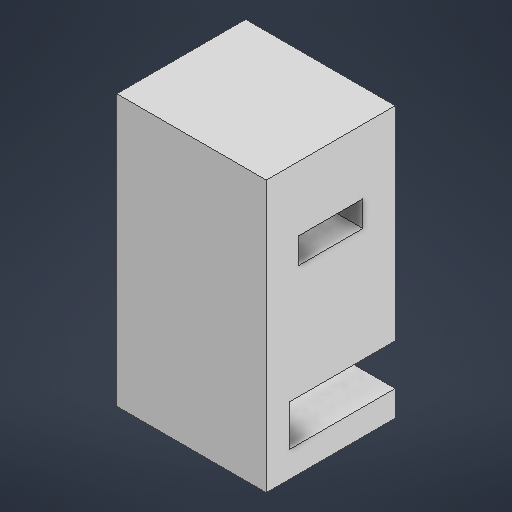
# Autodesk Inventor part: drone_battery_holder
Saved by Autodesk Inventor 2026.1 (Build 301233000, 233)
## iProperties
Created: 2025-08-09
Part Number: drone_battery_holder
Material: Generic
Document SubType Name: Modeling
Designer: rohit
Density: 1 g/cm^3
Appearance: Default
Author: rohit
Autodesk Inventor part; units mm, degrees
ref_plane "YZ Plane" through (0, 0, 0) normal (1, 0, 0) x (0, 1, 0)
ref_plane "XZ Plane" through (0, 0, 0) normal (0, 1, 0) x (-1, 0, 0)
ref_plane "XY Plane" through (0, 0, 0) normal (0, 0, 1) x (1, 0, 0)
sketch "Sketch1" plane through (0, 0, 0) normal (0, 1, 0) x (-1, 0, 0)
  line L0 (0, 0) -> (14.732, 0)
  line L1 (14.732, 0) -> (14.732, -12.7)
  line L2 (14.732, -12.7) -> (0, -12.7)
  line L3 (0, -12.7) -> (0, 0)
  dimension "d0" = 12.7
  dimension "d1" = 14.732
  constraints: 8 end point, 2 parallel, 1 horizontal, 1 perpendicular
  measures "d0" distance of L0.end L1.end
  measures "d1" distance of L1.end L2.end
extrude "Extrusion1" add sketch "Sketch1" along normal blind 26.67
sketch "Sketch2" plane through (0, 0, -12.7) normal (0, 0, -1) x (-1, 0, 0)
  line L0 (0, 0) -> (14.732, 0) projected
  line L1 (14.732, 0) -> (14.732, 2.54)
  line L2 (14.732, 0) -> (14.732, 26.67) projected
  line L3 (14.732, 2.54) -> (14.732, 6.604)
  line L4 (14.732, 6.604) -> (0, 6.604)
  line L5 (0, 0) -> (0, 26.67) projected
  line L6 (14.732, 2.54) -> (0, 2.54)
  line L7 (0, 2.54) -> (0, 6.604)
  line L8 (0, 6.604) -> (14.732, 6.604)
  line L9 (14.732, 6.604) -> (14.732, 2.54)
  dimension "d4" = 2.54
  dimension "d5" = 4.064
  constraints: 14 end point, 3 point on line, 2 horizontal, 2 parallel, 1 perpendicular
  measures "d4" distance of L0.end L1.end
  measures "d5" distance of L1.end L3.end
extrude "Extrusion2" cut sketch "Sketch2" against normal blind 10.414 contours L5 L4 L2 L6
sketch "Sketch3" plane through (0, 0, 0) normal (1, 0, 0) x (0, 0, -1)
  line L0 (0, 26.67) -> (12.7, 26.67) projected
  line L1 (0, 26.67) -> (6.35, 26.67)
  line L2 (6.35, 26.67) -> (6.35, 20.32)
  line L3 (6.35, 20.32) -> (3.175, 20.32)
  line L4 (3.175, 20.32) -> (3.175, 17.78)
  line L5 (3.175, 20.32) -> (9.525, 20.32)
  line L6 (9.525, 20.32) -> (9.525, 17.78)
  line L7 (9.525, 17.78) -> (3.175, 17.78)
  line L8 (3.175, 17.78) -> (3.175, 20.32)
  point P0 (0, 0)
  dimension "d8" = 6.35
  dimension "d9" = 6.35
  dimension "d10" = 3.175
  dimension "d11" = 2.54
  dimension "d12" = 6.35
  constraints: 16 end point, 4 perpendicular, 2 parallel, 1 horizontal, 1 midpoint
  measures "d8" distance of L0.start L1.end
  measures "d9" distance of L1.end L2.end
  measures "d10" distance of L2.end L3.end
  measures "d11" distance of L3.end L4.end
  measures "d12" distance of L6.end L7.end
extrude "Extrusion3" cut sketch "Sketch3" against normal blind 15.1765
body "Solid1"
